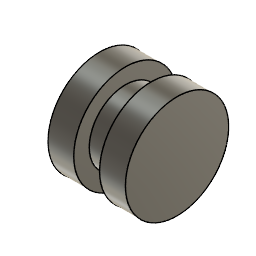
turning dan milling (Autodesk Fusion 360 design; units mm, degrees)
part number: 2026-06-24-22-54-10-954
Autodesk Fusion 360 part; units mm, degrees
sketch "Sketch1" plane through (0, 0, 0) normal (0, 0, 1) x (1, 0, 0)
  line L0 (0, 0) -> (0, -100)
  line L1 (0, -100) -> (-50, -100)
  line L2 (-100, -100) -> (-150, -100)
  line L3 (-150, -100) -> (-150, -50)
  line L4 (-150, -50) -> (-190, -30)
  line L5 (-190, -30) -> (-190, 0)
  line L6 (-190, 0) -> (0, 0)
  line L7 (-50, -100) -> (-50, -70)
  line L8 (-50, -70) -> (-100, -70)
  line L9 (-100, -70) -> (-100, -100)
  constraint coincident L0.start L6.end
  constraint vertical L0
  constraint perpendicular L0 L1
  constraint perpendicular L2 L3
  constraint perpendicular L2 L5
  constraint perpendicular L0 L6
  constraint perpendicular L1 L7
  constraint perpendicular L7 L8
  constraint perpendicular L2 L9
revolve "Revolve1" add sketch "Sketch1" angle 360 about axis through (-190, 0, 0) along (1, 0, 0)
